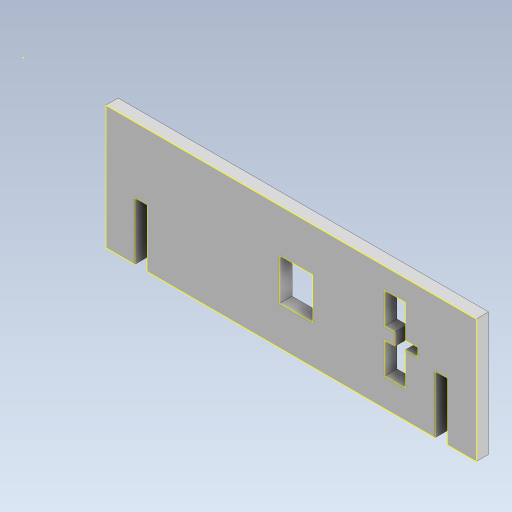
# Autodesk Inventor part: 零件8
Saved by Autodesk Inventor 2023 (Build 270158000, 158)
## iProperties
Created: 2023-05-16
Part Number: 零件8
Material: 一般
Document SubType Name: Modeling
Designer: Johnny Jou
Density: 1 g/cm^3
Appearance: 預設
Author: Johnny Jou
Autodesk Inventor part; units mm, degrees
ref_plane "YZ Plane" through (0, 0, 0) normal (1, 0, 0) x (0, 1, 0)
ref_plane "XZ Plane" through (0, 0, 0) normal (0, 1, 0) x (-1, 0, 0)
ref_plane "XY Plane" through (0, 0, 0) normal (0, 0, 1) x (1, 0, 0)
sketch "草圖1" plane through (0, 0, 0) normal (0, 0, 1) x (1, 0, 0)
  line L0 (0, 0) -> (130, 0)
  line L1 (130, 0) -> (130, -27)
  line L2 (130, -27) -> (0, -27)
  line L3 (0, -27) -> (0, 0)
  line L4 (27.05, -27) -> (30, -27)
  line L5 (30, -27) -> (30, -16)
  line L6 (30, -16) -> (27.05, -16)
  line L7 (27.05, -16) -> (27.05, -27)
  line L8 (100, -27) -> (102.95, -27)
  line L9 (102.95, -27) -> (102.95, -16)
  line L10 (102.95, -16) -> (100, -16)
  line L11 (100, -16) -> (100, -27)
  line L12 (30, -16) -> (100, -16)
  point P0 (65, -16)
  point P1 (65, -27)
  dimension "d0" = 70
  dimension "d1" = 130
  dimension "d2" = 2.95
  dimension "d3" = 2.95
  dimension "d4" = 11
  dimension "d5" = 27
  constraints: 26 end point, 6 parallel, 4 perpendicular, 4 point on line, 2 midpoint, 1 horizontal, 1 vertical alignment
  measures "d0" distance between parallel lines of L11 L5
  measures "d1" distance of L1.end L2.end
  measures "d2" distance of L9.end L10.end
  measures "d3" distance of L5.end L6.end
  measures "d4" distance of L6.end L4.start
  measures "d5" distance of L0.end L1.end
extrude "擠出1" add sketch "草圖1" along normal blind 3 contours L0 L1 L2 L9 L10 L12 L6 L7 L3 | L5 L12 L11 L2
sketch "草圖4" plane through (0, 0, 3) normal (0, 0, 1) x (1, 0, 0)
  line L0 (0, -27) -> (27.05, -27) projected
  line L1 (0, -27) -> (130, -27)
  line L2 (130, -27) -> (130, -30)
  line L3 (130, -30) -> (0, -30)
  line L4 (0, -30) -> (0, -27)
  line L5 (100, -27) -> (100, -16) projected
  line L6 (100, -27) -> (100, -30)
  line L7 (102.95, -16) -> (102.95, -27) projected
  line L8 (102.95, -27) -> (102.95, -30)
  line L9 (27.05, -27) -> (27.05, -30)
  line L10 (30, -27) -> (100, -27) projected
  line L11 (30, -27) -> (30, -30)
  line L12 (102.95, -27) -> (130, -27) projected
  line L13 (110, -27) -> (130, -27)
  line L14 (130, -27) -> (130, 0) projected
  dimension "d49" = 3
  constraints: 18 end point, 5 perpendicular, 5 point on line, 2 parallel, 1 collinear, 1 horizontal
  measures "d49" distance of L1.end L2.end
extrude "擠出4" add sketch "草圖4" against normal up to surface (3 mm away) contours L0 L9 L3 L4 | L1 L6 L3 L11 | L1 L2 L3 L8
sketch "草圖5" plane through (0, 0, 3) normal (0, 0, 1) x (1, 0, 0)
  line L0 (130, 0) -> (0, 0) projected
  line L1 (0, 0) -> (0, -30) projected
  line L2 (0, -30) -> (27.05, -30) projected
  line L3 (27.05, -30) -> (27.05, -16) projected
  line L4 (27.05, -16) -> (30, -16) projected
  line L5 (30, -16) -> (30, -30) projected
  line L6 (30, -30) -> (100, -30) projected
  line L7 (100, -30) -> (100, -16) projected
  line L8 (100, -16) -> (102.95, -16) projected
  line L9 (102.95, -16) -> (102.95, -30) projected
  line L10 (102.95, -30) -> (130, -30) projected
  line L11 (130, -30) -> (130, 0) projected
  line L12 (130, -30) -> (102.95, -30) projected
  line L13 (130, 0) -> (110, 0)
  line L14 (110, 0) -> (110, -30)
  line L15 (110, -30) -> (130, -30)
  line L16 (130, -30) -> (130, 0)
  line L17 (0, -30) -> (0, 0)
  line L18 (0, 0) -> (20, 0)
  line L19 (20, 0) -> (20, -30)
  line L20 (20, -30) -> (0, -30)
  point P0 (130, -15)
  dimension "d33" = 20
  dimension "d51" = 20
  constraints: 16 end point, 4 parallel, 3 perpendicular, 1 horizontal, 1 midpoint, 1 point on line
  measures "d33" distance from line of point (130, -15) L14
  measures "d51" distance between parallel lines of L1 L19
extrude "擠出5" cut sketch "草圖5" against normal up to surface (3 mm away) contours L11 L10 L14 L0 | L19 L2 L1 L0
sketch "草圖7" plane through (0, 0, 3) normal (0, 0, 1) x (1, 0, 0)
  line L0 (90.25, -5.137) -> (90.25, -23.137)
  line L1 (90.25, -23.137) -> (92.75, -23.137)
  line L2 (92.75, -23.137) -> (92.75, -5.137)
  line L3 (92.75, -5.137) -> (90.25, -5.137)
  line L4 (100, -30) -> (100, -16) projected
  line L5 (100, -16) -> (102.95, -16) projected
  line L6 (90.25, -5.137) -> (90.25, -12.637)
  line L7 (90.25, -12.637) -> (87.75, -12.637)
  line L8 (87.75, -12.637) -> (87.75, -5.137)
  line L9 (87.75, -5.137) -> (90.25, -5.137)
  line L10 (90.25, -15.637) -> (90.25, -23.137)
  line L11 (90.25, -23.137) -> (87.75, -23.137)
  line L12 (87.75, -23.137) -> (87.75, -15.637)
  line L13 (87.75, -15.637) -> (90.25, -15.637)
  line L14 (92.75, -15.137) -> (95.75, -15.137)
  line L15 (95.75, -15.137) -> (95.75, -13.137)
  line L16 (95.75, -13.137) -> (92.75, -13.137)
  line L17 (92.75, -13.137) -> (92.75, -15.137)
  line L18 (102.95, -5.137) -> (102.95, -23.137)
  line L19 (102.95, -23.137) -> (105.45, -23.137)
  line L20 (105.45, -23.137) -> (105.45, -5.137)
  line L21 (105.45, -5.137) -> (102.95, -5.137)
  line L22 (102.95, -16) -> (102.95, -30) projected
  line L23 (30, -30) -> (100, -30) projected
  line L24 (62.25, -10.5805) -> (70.25, -10.5805)
  line L25 (70.25, -10.5805) -> (70.25, -20.5805)
  line L26 (70.25, -20.5805) -> (62.25, -20.5805)
  line L27 (62.25, -20.5805) -> (62.25, -10.5805)
  point P0 (0, 0)
  point P1 (91.5, -5.137)
  point P2 (95.75, -14.137)
  point P3 (92.75, -14.137)
  point P4 (66.25, -20.5805)
  dimension "d36" = 7.25
  dimension "d37" = 2.5
  dimension "d38" = 18
  dimension "d40" = 18
  dimension "d41" = 2.5
  dimension "d42" = 7.5
  dimension "d43" = 7.5
  dimension "d44" = 2.5
  dimension "d45" = 2
  dimension "d46" = 3
  dimension "d50" = 6.863
  dimension "d52" = 10
  dimension "d53" = 8
  dimension "d54" = 20
  constraints: 48 end point, 13 parallel, 7 perpendicular, 7 point on line, 4 midpoint, 3 collinear, 1 horizontal, 1 horizontal alignment
  measures "d36" distance between parallel lines of L4 L2
  measures "d37" distance between parallel lines of L2 L0
  measures "d38" distance of L0.start L0.end
  measures "d40" distance of L19.end L20.end
  measures "d41" distance of L6.end L7.end
  measures "d42" distance of L7.end L8.end
  measures "d43" distance of L11.end L12.end
  measures "d44" distance between parallel lines of L18 L20
  measures "d45" distance of L14.end L15.end
  measures "d46" distance of L15.end L16.end
  measures "d50" distance between parallel lines of L23 L1
  measures "d52" distance from line of L24 point (66.25, -20.581)
  measures "d53" distance of L24.start L24.end
  measures "d54" distance between parallel lines of L0 L25
extrude "擠出6" cut sketch "草圖7" against normal up to surface (3 mm away) contours L3 L2 L1 L0 | L0 L7 L8 L9 | L0 L11 L12 L13 | L16 L15 L14 L2 | L24 L25 L26 L27
sketch "草圖9" plane through (0, 0, 3) normal (0, 0, 1) x (1, 0, 0)
  line L0 (102.95, -16) -> (102.95, -30) projected
  line L1 (102.95, -30) -> (110, -30) projected
  line L2 (110, -30) -> (110, 0) projected
  line L3 (110, 0) -> (20, 0) projected
  line L4 (20, 0) -> (20, -30) projected
  line L5 (20, -30) -> (27.05, -30) projected
  line L6 (27.05, -30) -> (27.05, -16) projected
  line L7 (27.05, -16) -> (30, -16) projected
  line L8 (30, -16) -> (30, -30) projected
  line L9 (30, -30) -> (100, -30) projected
  line L10 (100, -30) -> (100, -16) projected
  line L11 (100, -16) -> (102.95, -16) projected
  line L12 (95.75, -15.137) -> (92.75, -15.137) projected
  line L13 (92.75, -15.137) -> (92.75, -23.137) projected
  line L14 (92.75, -23.137) -> (87.75, -23.137) projected
  line L15 (87.75, -23.137) -> (87.75, -15.637) projected
  line L16 (87.75, -15.637) -> (90.25, -15.637) projected
  line L17 (90.25, -15.637) -> (90.25, -12.637) projected
  line L18 (90.25, -12.637) -> (87.75, -12.637) projected
  line L19 (87.75, -12.637) -> (87.75, -5.137) projected
  line L20 (87.75, -5.137) -> (92.75, -5.137) projected
  line L21 (92.75, -5.137) -> (92.75, -13.137) projected
  line L22 (92.75, -13.137) -> (95.75, -13.137) projected
  line L23 (95.75, -13.137) -> (95.75, -15.137) projected
  line L24 (70.25, -20.5805) -> (62.25, -20.5805) projected
  line L25 (62.25, -20.5805) -> (62.25, -10.5805) projected
  line L26 (62.25, -10.5805) -> (70.25, -10.5805) projected
  line L27 (70.25, -10.5805) -> (70.25, -20.5805) projected
  point P0 (0, 0)
